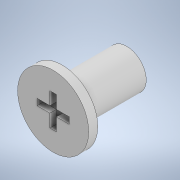
# Autodesk Inventor part: CSPELH-SUS-M3-5
Saved by Autodesk Inventor 2020 (Build 240168000, 168)
## iProperties
Created: 2020-06-27
Part Number: CSPELH-SUS-M3-5
Material: 一般
Document SubType Name: Modeling
Designer: haya
Density: 1 g/cm^3
Appearance: 既定
Author: haya
Autodesk Inventor part; units mm, degrees
ref_plane "YZ Plane" through (0, 0, 0) normal (1, 0, 0) x (0, 1, 0)
ref_plane "XZ Plane" through (0, 0, 0) normal (0, 1, 0) x (-1, 0, 0)
ref_plane "XY Plane" through (0, 0, 0) normal (0, 0, 1) x (1, 0, 0)
sketch "スケッチ1" plane through (0, 0, 0) normal (0, 0, 1) x (1, 0, 0)
  circle A0 centre (0, 0) radius 2.75
  dimension "d0" = 5.5
  constraints: 1 centre point, 1 coincident
  measures "d0" diameter of A0
extrude "押し出し1" add sketch "スケッチ1" along normal blind 0.7
sketch "スケッチ2" plane through (0, 0, 0) normal (0, 0, -1) x (-1, 0, 0)
  circle A0 centre (0, 0) radius 1.5
  dimension "d3" = 3
  constraints: 1 centre point, 1 coincident
  measures "d3" diameter of A0
extrude "押し出し2" add sketch "スケッチ2" along normal blind 5
sketch "スケッチ3" plane through (0, 0, 0.7) normal (0, 0, 1) x (1, 0, 0)
  line L0 (-1.25, 0.25) -> (1.25, 0.25)
  line L1 (1.25, 0.25) -> (1.25, -0.25)
  line L2 (1.25, -0.25) -> (-1.25, -0.25)
  line L3 (-1.25, -0.25) -> (-1.25, 0.25)
  line L4 (-0.25, 1.25) -> (0.25, 1.25)
  line L5 (0.25, 1.25) -> (0.25, -1.25)
  line L6 (0.25, -1.25) -> (-0.25, -1.25)
  line L7 (-0.25, -1.25) -> (-0.25, 1.25)
  line L8 (0, 0) -> (0, 1.7976)
  line L9 (0, 0) -> (2.75, 0)
  circle A0 centre (0, 0) radius 2.75 projected
  point P0 (-0.25, 0.25)
  point P1 (-0.25, -0.25)
  point P2 (0.25, -0.25)
  point P3 (0.25, 0.25)
  dimension "d6" = 0.5
  dimension "d7" = 0.5
  dimension "d8" = 2.5
  dimension "d9" = 2.5
  constraints: 20 end point, 4 parallel, 3 horizontal, 2 perpendicular, 1 horizontal alignment, 1 vertical, 5 other
  measures "d6" distance of L0.end L1.end
  measures "d7" distance of L4.start L4.end
  measures "d8" distance of L6.end L4.start
  measures "d9" distance of L1.end L2.end
extrude "押し出し3" cut sketch "スケッチ3" against normal blind 0.5 contours L0 L7 L2 L3 | L7 L4 L8 L0 | L0 L8 L9 L5 L2 L7 | L8 L4 L5 L0 | L0 L5 L9 L8 | L2 L5 L6 L7 | L0 L1 L9 L5 | L5 L9 L1 L2
